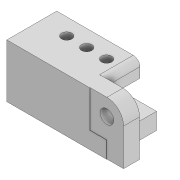
# Autodesk Inventor part: Bending_hinge
Saved by Autodesk Inventor 2022 (Build 260153000, 153)
## iProperties
Created: 2022-07-29
Part Number: Bending_hinge
Material: Generic
Document SubType Name: Modeling
Designer: dell
Density: 1 g/cm^3
Appearance: Default
Author: dell
Autodesk Inventor part; units mm, degrees
ref_plane "YZ Plane" through (0, 0, 0) normal (1, 0, 0) x (0, 1, 0)
ref_plane "XZ Plane" through (0, 0, 0) normal (0, 1, 0) x (-1, 0, 0)
ref_plane "XY Plane" through (0, 0, 0) normal (0, 0, 1) x (1, 0, 0)
sketch "Sketch2" plane through (0, 0, 0) normal (0, 1, 0) x (-1, 0, 0)
  line L0 (0, 0) -> (30, 0)
  line L1 (30, 0) -> (30, -10)
  line L2 (30, -10) -> (0, -10)
  line L3 (0, -10) -> (0, 0)
  circle A0 centre (10, -5) radius 1.55
  dimension "d0" = 3.1
  dimension "d1" = 10
  dimension "d2" = 5
  dimension "d3" = 30
  dimension "d4" = 10
  constraints: 8 end point, 2 parallel, 1 centre point, 1 horizontal, 1 perpendicular
  measures "d0" diameter of A0
  measures "d1" distance from line of L3 A0.centre
  measures "d2" distance from line of L0 A0.centre
  measures "d3" distance between parallel lines of L3 L1
  measures "d4" distance between parallel lines of L0 L2
extrude "Extrusion1" add sketch "Sketch2" along normal blind 5 contours L0 L1 L2 L3 | A0
extrude "Extrusion2" cut sketch "Sketch2" along normal blind 10 contours A0
pattern_linear "Rectangular Pattern1" count 3 spacing 6 along (-1, 0, 0) of "Extrusion2"
pattern_linear "Rectangular Pattern2" count 2 spacing 11.1 along (0, -1, 0) of "Extrusion1", "Extrusion2", "Rectangular Pattern1"
sketch "Sketch3" plane through (-30, 0, 0) normal (0, 0, 1) x (1, 0, 0)
  line L0 (0, 0) -> (0, 5) projected
  line L1 (0, 5) -> (30, 5) projected
  line L2 (30, 5) -> (30, 0) projected
  line L3 (30, 0) -> (0, 0) projected
  line L4 (0, -11.1) -> (0, -6.1) projected
  line L5 (0, -6.1) -> (30, -6.1) projected
  line L6 (30, -6.1) -> (30, -11.1) projected
  line L7 (30, -11.1) -> (0, -11.1) projected
  line L8 (0, 5) -> (30, 5) projected
  line L9 (0, 5) -> (30, 5)
  line L10 (30, 5) -> (30, -11.1)
  line L11 (30, -11.1) -> (0, -11.1)
  line L12 (0, -11.1) -> (0, 5)
  line L13 (0, 0) -> (30, 0) projected
  circle A0 centre (30, 0) radius 2.05
  line L14 (25, 5) -> (35, 5)
  line L15 (35, 5) -> (35, -11.1)
  line L16 (35, -11.1) -> (25, -11.1)
  line L17 (25, -11.1) -> (25, 5)
  line L18 (0, -11.1) -> (30, -11.1) projected
  point P0 (30, 2.05)
  point P1 (30, -2.05)
  dimension "d28" = 4.1
  dimension "d29" = 10
  dimension "d31" = 5
  constraints: 16 end point, 4 parallel, 2 collinear, 2 horizontal, 2 perpendicular, 1 centre point, 1 coincident
  measures "d28" diameter of A0
  measures "d29" distance of L15.end L16.end
  measures "d31" distance from line of L2.end L17
extrude "Extrusion3" add sketch "Sketch3" along normal blind 5 contours L0 L1 L17 L3 | L3 L17 L5 L12 | L17 L1 L2 A0 L3 | L3 A0 L10 L5 L17 | L5 L17 L7 L4 | A0 L2 L3 | L3 L10 A0 | L5 L6 L7 L17
extrude "Extrusion4" add sketch "Sketch3" along normal blind 5 contours L14 L15 L16 L6 L10 A0 L2
extrude "Extrusion5" cut sketch "Sketch3" along normal mid plane 100 contours A0 L2 L3 | L3 L10 A0
sketch "Sketch4" plane through (0, 5, -10) normal (0, 0, -1) x (-1, 0, 0)
  line L0 (0, 0) -> (5, 0)
  line L1 (5, 0) -> (5, -5)
  line L2 (5, -5) -> (0, -5)
  line L3 (0, -5) -> (0, 0)
  line L4 (2.05, -5) -> (30, -5) projected
  point P0 (0, -5)
  dimension "d32" = 5
  constraints: 8 end point, 2 parallel, 1 collinear, 1 horizontal, 1 perpendicular
  measures "d32" distance between parallel lines of L1 L3
extrude "Extrusion6" cut sketch "Sketch4" against normal blind 10
fillet "Fillet1" radius 5 1 edges at (5, 5, 2.5)
sketch "Sketch5" plane through (-30, 0, 0) normal (0, 0, -1) x (-1, 0, 0)
  arc A0 (-30, 5) -> (-35, 0) centre (-30, 0) ccw projected
  line L0 (-35, -11.1) -> (-35, 0) projected
  line L1 (-30, -11.1) -> (-35, -11.1) projected
  line L2 (-30, -6.1) -> (-30, -11.1) projected
  line L3 (0, -6.1) -> (-30, -6.1) projected
  line L4 (0, 0) -> (0, -6.1) projected
  line L5 (0, 0) -> (-25, 0) projected
  line L6 (-25, 5) -> (-25, 0) projected
  line L7 (-30, 5) -> (-25, 5) projected
  circle A1 centre (-30, 0) radius 2.05 projected
  line L8 (-25, 0) -> (-25, -6.1)
  line L9 (0, -6.1) -> (-30, -6.1) projected
  constraints: 2 end point, 1 point on line, 1 vertical
extrude "Extrusion7" cut sketch "Sketch5" against normal blind 0.1 contours L7 L6 L8 L3 L2 L1 L0 A0
sketch "Sketch6" plane through (-30, 0, 5) normal (0, 0, 1) x (1, 0, 0)
  line L0 (25, -6.1) -> (30, -6.1) projected
  line L1 (25, 5) -> (25, -6.1) projected
  line L2 (30, 5) -> (25, 5) projected
  arc A0 (35, 0) -> (30, 5) centre (30, 0) ccw projected
  line L3 (35, -11.1) -> (35, 0) projected
  line L4 (30, -11.1) -> (35, -11.1) projected
  line L5 (30, -6.1) -> (30, -11.1) projected
  circle A1 centre (30, 0) radius 2.05 projected
extrude "Extrusion8" cut sketch "Sketch6" against normal blind 0.1
fillet "Fillet2" radius 2 1 edges at (-5, 5, -4.95)
body "Solid1"
